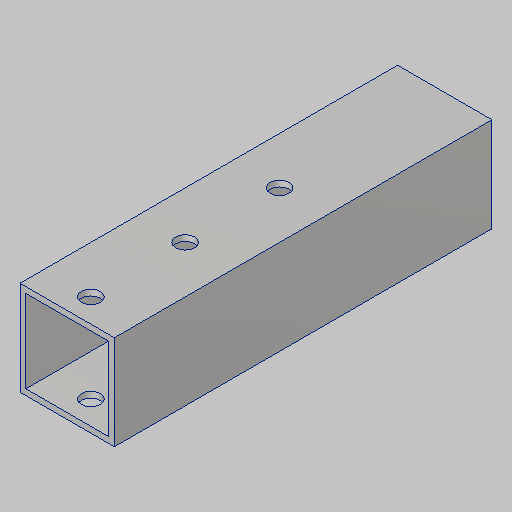
# Autodesk Inventor part: DB1-012
Saved by Autodesk Inventor 2023.5 (Build 275446000, 446)
## iProperties
Created: 2025-01-14
Part Number: DB1-012
Material: Aluminum 6061
Document SubType Name: Modeling
Designer: mavericks
Density: 2.7 g/cm^3
Appearance: Aluminum - Flat
Author: mavericks
Autodesk Inventor part; units mm, degrees
ref_plane "YZ Plane" through (0, 0, 0) normal (1, 0, 0) x (0, 1, 0)
ref_plane "XZ Plane" through (0, 0, 0) normal (0, 1, 0) x (-1, 0, 0)
ref_plane "XY Plane" through (0, 0, 0) normal (0, 0, 1) x (1, 0, 0)
sketch "Sketch1" plane through (0, 0, 0) normal (0, 0, 1) x (1, 0, 0)
  line L0 (-12.7, -12.7) -> (12.7, -12.7)
  line L1 (12.7, -12.7) -> (12.7, 12.7)
  line L2 (12.7, 12.7) -> (-12.7, 12.7)
  line L3 (-12.7, 12.7) -> (-12.7, -12.7)
  line L4 (-12.7, -12.7) -> (12.7, 12.7) construction
  line L5 (12.7, -12.7) -> (-12.7, 12.7) construction
  line L6 (11.1125, -11.1125) -> (-11.1125, -11.1125)
  line L7 (-11.1125, -11.1125) -> (-11.1125, 11.1125)
  line L8 (-11.1125, 11.1125) -> (11.1125, 11.1125)
  line L9 (11.1125, 11.1125) -> (11.1125, -11.1125)
  line L10 (11.1125, -11.1125) -> (-11.1125, 11.1125) construction
  line L11 (-11.1125, -11.1125) -> (11.1125, 11.1125) construction
  point P0 (0, 0)
  dimension "d0" = 25.4
  dimension "d1" = 25.4
  dimension "d3" = 22.225
  dimension "d4" = 22.225
  constraints: 24 end point, 4 parallel, 3 midpoint, 2 horizontal, 2 perpendicular
  measures "d0" distance of L2.end L1.end
  measures "d1" distance of L1.end L0.end
  measures "d3" distance of L7.end L8.end
  measures "d4" distance of L6.end L7.end
extrude "Extrusion1" add sketch "Sketch1" along normal mid plane 101.6
sketch "Sketch2" plane through (-12.7, 12.7, 50.8) normal (0, 1, 0) x (1, 0, 0)
  line L0 (25.4, 0) -> (0, 0) projected
  point P0 (12.7, 50.8)
  point P1 (12.7, 6.35)
  point P2 (12.7, 31.75)
  point P3 (12.7, 57.15)
  point P4 (12.7, 0)
  point P5 (12.7, 0)
  dimension "d7" = 6.35
  dimension "d8" = 25.4
  dimension "d9" = 25.4
  constraints: 3 vertical alignment, 2 midpoint
  measures "d7" distance of point (12.7, 0) point (12.7, 6.35)
  measures "d8" distance of point (12.7, 6.35) point (12.7, 31.75)
  measures "d9" distance of point (12.7, 57.15) point (12.7, 31.75)
hole "Hole1" at (0, 12.7, 44.45) at (0, 12.7, 19.05) at (0, 12.7, -6.35) direction (0, -1, 0) diameter 5.1054 end through all clearance for "Flat Head Machine Screw (82)" size "#10" standard "Ansi Unified Screw Threads"
body "Solid1"
